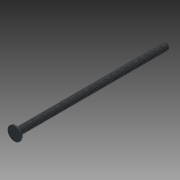
# Autodesk Inventor part: rod
Saved by Autodesk Inventor 2015 (Build 190159000, 159)
## iProperties
Created: 2015-03-27
Part Number: rod
Material: Steel
Document SubType Name: Modeling
Designer: 23902
Density: 7.85 g/cm^3
Appearance: Iron Gray
Mass: 23.7367 g
Surface Area: 25.4469 cm^2
Volume: 3.02378 cm^3
Author: 23902
Autodesk Inventor part; units mm, degrees
ref_plane "YZ Plane" through (0, 0, 0) normal (1, 0, 0) x (0, 1, 0)
ref_plane "XZ Plane" through (0, 0, 0) normal (0, 1, 0) x (-1, 0, 0)
ref_plane "XY Plane" through (0, 0, 0) normal (0, 0, 1) x (1, 0, 0)
sketch "Sketch1" plane through (0, 0, 0) normal (0, 1, 0) x (-1, 0, 0)
  line L0 (-9.9492, -0.156) -> (-3.4492, -0.156)
  circle A0 centre (-3.4492, -0.156) radius 5
  point P0 (0, 0)
  dimension "d10" = 10
  constraints: 2 end point, 1 centre point, 1 coincident, 1 horizontal
  measures "d10" diameter of A0
extrude "Extrusion1" add sketch "Sketch1" along normal blind 1
sketch "Sketch2" plane through (0, 1, 0) normal (0, 1, 0) x (1, 0, 0)
  line L0 (-3.0508, -6.344) -> (9.9492, -6.344) projected
  circle A0 centre (3.4492, 0.156) radius 2.5
  point P0 (0, 0)
  dimension "d5" = 5
  constraints: 1 centre point
  measures "d5" diameter of A0
extrude "Extrusion2" add sketch "Sketch2" along normal blind 110
thread "Thread1" size "M5x0.8" class "6g" standard "ANSI Metric M Profile" full length
body "Solid1"
